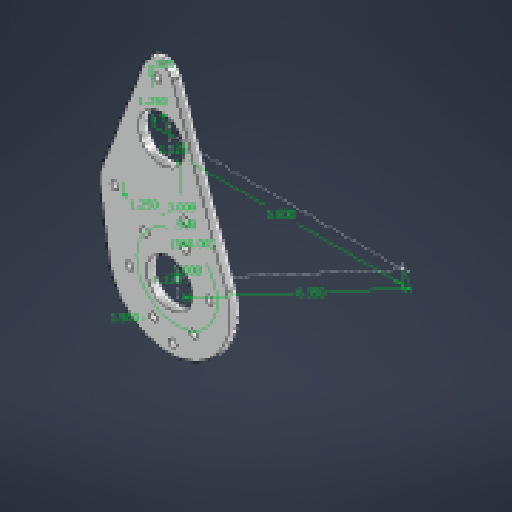
# Autodesk Inventor part: PLATE,TURRET,MOTOR,MOUNT
Saved by Autodesk Inventor 2026 (Build 300175000, 175)
## iProperties
Created: 2026-02-09
Part Number: PLATE,TURRET,MOTOR,MOUNT
Material: Aluminum 6061
Document SubType Name: Sheet Metal
Designer: littl
Density: 2.7 g/cm^3
Sheet Metal Rule: Default
Appearance: Aluminum - Flat
Author: littl
Autodesk Inventor part; units mm, degrees
ref_plane "YZ Plane" through (0, 0, 0) normal (1, 0, 0) x (0, 1, 0)
ref_plane "XZ Plane" through (0, 0, 0) normal (0, 1, 0) x (-1, 0, 0)
ref_plane "XY Plane" through (0, 0, 0) normal (0, 0, 1) x (1, 0, 0)
sketch "Sketch2" plane through (0, 0, 0) normal (0, 0, 1) x (1, 0, 0)
  circle A0 centre (0, 0) radius 14.2875
  circle A1 centre (-5.0745, 76.0308) radius 14.2875
  line L0 (142.2455, 76.0308) -> (0, 0) construction
  line L1 (142.2455, 76.0308) -> (-5.0745, 76.0308) construction
  line L2 (-5.0745, 76.0308) -> (0, 0) construction
  line L3 (-7.1889, 107.7104) -> (-5.0745, 76.0308) construction
  line L4 (0, 0) -> (2.5373, -38.0154) construction
  line L5 (10.1345, 38.8612) -> (-2.5373, 38.0154) construction
  line L6 (-34.2168, 35.901) -> (-2.5373, 38.0154) construction
  arc A2 (1.5986, 111.3853) -> (-16.1034, 111.0656) centre (-7.1889, 107.7104) ccw
  arc A3 (-43.1313, 39.2563) -> (-43.7399, 36.0907) centre (-34.2168, 35.901) ccw
  line L7 (1.5986, 111.3853) -> (41.0083, 17.1499)
  line L8 (-16.1034, 111.0656) -> (-43.1313, 39.2563)
  arc A4 (-44.4412, 0.8853) -> (41.0083, 17.1499) centre (0, 0) ccw
  line L9 (-44.4412, 0.8853) -> (-43.7399, 36.0907)
  line L10 (0, 0) -> (-24.5345, 6.574) construction
  line L11 (0, 0) -> (-29.6173, 0) construction
  point P0 (24.5345, -6.574)
  point P1 (17.9605, 17.9605)
  point P2 (-6.574, 24.5345)
  point P3 (-17.9605, -17.9605)
  point P4 (6.574, -24.5345)
  dimension "d40" = 28.575
  dimension "d43" = 360
  dimension "d45" = 25.4
  dimension "d46" = 28.575
  dimension "d47" = 76.2
  dimension "d48" = 161.29
  dimension "d49" = 147.32
  dimension "d50" = 31.75
  dimension "d51" = 12.7
  dimension "d52" = 31.75
  dimension "d53" = 9.525
  dimension "d56" = 44.45
  dimension "d65" = 15
  dimension "d73" = 38.1
  constraints: 24 end point, 6 point on circle, 6 tangent, 5 centre point, 4 coincident, 3 collinear, 2 horizontal, 1 equal radius, 1 midpoint, 1 perpendicular, 7 other
  measures "d40" diameter of A0
  measures "d45" distance of point (24.535, -6.574) point (0, 0)
  measures "d46" diameter of A1
  measures "d47" distance of point (0, 0) L1.end
  measures "d48" distance of point (0, 0) L0.start
  measures "d49" distance of L1.end L0.start
  measures "d50" distance of L3.start L1.end
  measures "d51" distance of L5.start L5.end
  measures "d52" distance of L6.start L5.end
  measures "d53" radius of A2
  measures "d56" radius of A4
  measures "d65" angle of L10 L11
  measures "d73" distance of L0.end L4.end
extrude "Plate2" add sketch "Sketch2" along normal blind 4.7625
hole "Hole3" at (17.9605, 17.9605, 0) at (-17.9605, -17.9605, 0) at (142.2455, 76.0308, 0) at (-6.574, 24.5345, 0) at (6.574, -24.5345, 0) direction (0, 0, 1) diameter 4.9784 end through all clearance for "Flat Head Machine Screw (82)" size "#10" standard "Ansi Unified Screw Threads"
hole "Hole4" at (10.1345, 38.8612, 0) at (-34.2168, 35.901, 0) at (-7.1889, 107.7104, 0) at (2.5373, -38.0154, 0) direction (0, 0, 1) diameter 6.5278 end through all clearance for "Flat Head Machine Screw (82)" size "1/4" standard "Ansi Unified Screw Threads"
equation "\"BendRadius\" = Thickness"
equation "\"BendReliefWidth\" = Thickness"
equation "\"BendReliefDepth\" = 0.5 * Thickness"
equation "\"CornerReliefSize\" = 4 * Thickness"
equation "\"MinimumRemnant\" = 2 * Thickness"
equation "\"TransitionRadius\" = BendRadius"
equation "\"JacobiRadiusSize\" = BendRadius"
equation "\"GapSize\" = Thickness"
equation "\"Thickness\" = 4.7625"
body "Solid2"
